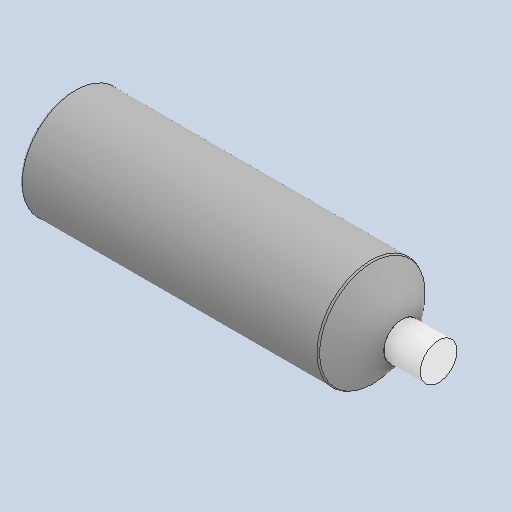
# Autodesk Inventor part: roller-Base-v1-petbottle
Saved by Autodesk Inventor 2025.2 (Build 292293000, 293)
## iProperties
Created: 2024-03-21
Part Number: roller-Base-v1-petbottle
Material: PET プラスチック
Document SubType Name: Modeling
Designer: haruy
Density: 1.541 g/cm^3
Appearance: 淡い灰色
Author: haruy
Autodesk Inventor part; units mm, degrees
ref_plane "YZ Plane" through (0, 0, 0) normal (1, 0, 0) x (0, 1, 0)
ref_plane "XZ Plane" through (0, 0, 0) normal (0, 1, 0) x (-1, 0, 0)
sketch "スケッチ4" plane through (0, 0, 0) normal (1, 0, 0) x (0, 1, 0)
  circle A0 centre (0, 0) radius 44
  circle A1 centre (0, 0) radius 42
  dimension "d6" = 88
  dimension "d7" = 2
  constraints: 2 centre point, 1 coincident
  measures "d6" diameter of A0
  measures "d7" radial gap between concentric circles of A0 A1
extrude "押し出し3" add sketch "スケッチ4" along normal blind 220
ref_plane "作業平面1" through (245, 0, 0) normal (1, 0, 0) x (0, 0, -1)
sketch "スケッチ5" plane through (245, 0, 0) normal (1, 0, 0) x (0, 0, -1)
  circle A0 centre (0, 0) radius 15
  circle A1 centre (0, 0) radius 13
  dimension "d11" = 30
  dimension "d12" = 2
  constraints: 2 centre point, 1 coincident
  measures "d11" diameter of A0
  measures "d12" radial gap between concentric circles of A0 A1
extrude "押し出し4" add sketch "スケッチ5" along normal blind 30 separate body
sketch "スケッチ6" plane through (275, 0, 0) normal (1, 0, 0) x (0, 0, -1)
  circle A0 centre (0, 0) radius 15
  constraints: 1 centre point, 1 coincident
extrude "押し出し5" add sketch "スケッチ6" against normal blind 2 bodies 2
loft "ロフト2" add bodies 1 section 1 edges at (220, -44, 0) section 2 edges at (245, 0, 15)
fillet "フィレット1" radius 2 1 edges at (220, -44, 0)
sketch "スケッチ7" plane through (0, 0, 0) normal (-1, 0, 0) x (0, 0, 1)
  circle A0 centre (0, 0) radius 44
  circle A1 centre (0, 0) radius 42
  constraints: 2 centre point, 2 coincident
extrude "押し出し6" add sketch "スケッチ7" along normal blind 25 bodies 1
sketch "スケッチ8" plane through (-25, 0, 0) normal (-1, 0, 0) x (0, 0, 1)
  circle A0 centre (0, 0) radius 44
  constraints: 1 centre point, 1 coincident
extrude "押し出し7" add sketch "スケッチ8" against normal blind 2 bodies 1
fillet "フィレット2" radius 2 1 edges at (-25, 0, -44)
